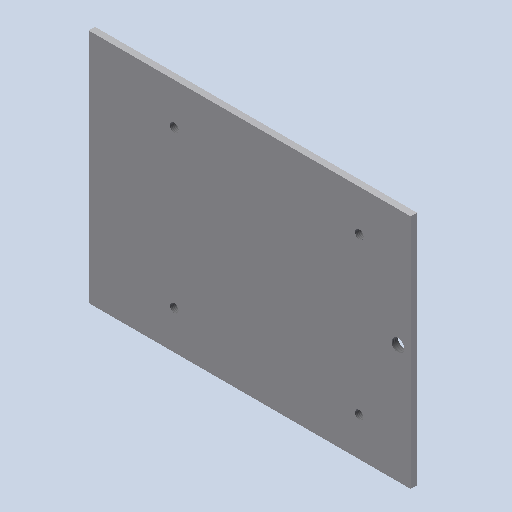
# Autodesk Inventor part: Tapa raspberry
Saved by Autodesk Inventor 2023 (Build 270158000, 158)
## iProperties
Created: 2022-11-11
Part Number: Tapa raspberry
Material: ABS Plastic
Document SubType Name: Modeling
Designer: Lenovo
Density: 1.06 g/cm^3
Appearance: Smooth - White
Author: Lenovo
Autodesk Inventor part; units mm, degrees
ref_plane "YZ Plane" through (0, 0, 0) normal (1, 0, 0) x (0, 1, 0)
ref_plane "XZ Plane" through (0, 0, 0) normal (0, 1, 0) x (-1, 0, 0)
ref_plane "XY Plane" through (0, 0, 0) normal (0, 0, 1) x (1, 0, 0)
sketch "Sketch1" plane through (0, 0, 0) normal (0, 0, 1) x (1, 0, 0)
  line L0 (0, 0) -> (93, 0)
  line L1 (93, 0) -> (93, 66)
  line L2 (93, 66) -> (0, 66)
  line L3 (0, 66) -> (0, 0)
  dimension "d0" = 93
  dimension "d1" = 66
  constraints: 8 end point, 2 parallel, 1 horizontal, 1 perpendicular
  measures "d0" distance of L2.end L1.end
  measures "d1" distance of L1.end L0.end
extrude "Extrusion1" add sketch "Sketch1" along normal blind 2
sketch "Sketch2" plane through (0, 0, 2) normal (0, 0, 1) x (1, 0, 0)
  line L0 (93, 0) -> (93, 66) projected
  line L1 (93, 66) -> (0, 66) projected
  line L2 (0, 66) -> (0, 0) projected
  line L3 (0, 0) -> (93, 0) projected
  line L4 (0, 70) -> (101, 70)
  line L5 (101, 70) -> (101, -4)
  line L6 (101, -4) -> (0, -4)
  line L7 (0, 66) -> (0, 70)
  line L8 (0, -4) -> (0, 0)
  dimension "d4" = 4
  dimension "d5" = 8
  dimension "d6" = 4
  constraints: 10 end point, 1 collinear, 1 point on line, 1 vertical
  measures "d4" distance between parallel lines of L1 L4
  measures "d5" distance between parallel lines of L0 L5
  measures "d6" distance between parallel lines of L6 L3
extrude "Extrusion2" add sketch "Sketch2" along normal blind 2
sketch "Sketch3" plane through (0, 0, 0) normal (0, 0, -1) x (-1, 0, 0)
  circle A0 centre (-26.8923, 57.0496) radius 1.375 projected
  circle A1 centre (-84.8923, 57.0496) radius 1.375 projected
  circle A2 centre (-84.8923, 8.0496) radius 1.375 projected
  circle A3 centre (-26.8923, 8.0496) radius 1.375 projected
  point P0 (0, 0)
hole "Hole1" at (26.8923, 57.0496, 0) at (84.8923, 57.0496, 0) at (84.8923, 8.0496, 0) at (26.8923, 8.0496, 0) direction (0, 0, 1) diameter 2.75 depth 4
sketch "Sketch4" plane through (0, 0, 4) normal (0, 0, 1) x (1, 0, 0)
  line L0 (101, 70) -> (0, 70) projected
  line L1 (0, -4) -> (101, -4) projected
  line L2 (0, 70) -> (0, -4) projected
  line L3 (101, -4) -> (101, 70) projected
  point P0 (0, 0)
  point P1 (97, 33)
  dimension "d16" = 37
  dimension "d18" = 4
  measures "d16" distance from line of point (97, 33) L0
  measures "d18" distance from line of L3 point (97, 33)
hole "Hole2" at (97, 33, 4) direction (0, 0, -1) diameter 4 depth 3
thread "Thread1" size "M4x0.7" class "6H" standard "ANSI Metric M Profile" full length
thread "Thread2" size "M3x0.5" class "6H" standard "ANSI Metric M Profile" full length
thread "Thread3" size "M3x0.5" class "6H" standard "ANSI Metric M Profile" full length
thread "Thread4" size "M3x0.5" class "6H" standard "ANSI Metric M Profile" full length
thread "Thread5" size "M3x0.5" class "6H" standard "ANSI Metric M Profile" full length
body "Solid1"
